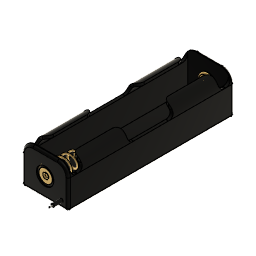
18650 battery holder (Autodesk Fusion 360 design; units mm, degrees)
Autodesk Fusion 360 part; units mm, degrees
note: some values were not read from the file. Set by a fixed rule: which face or edge a step refers to.
sketch "Esquisse1" plane through (0, 0, 0) normal (0, 1, 0) x (1, 0, 0)
  line L0 (-10.6, 9.1) -> (10.6, 9.1)
  line L1 (10.6, 9.1) -> (10.6, -4.1)
  line L2 (5.6, -9.1) -> (-5.6, -9.1)
  line L3 (-10.6, -4.1) -> (-10.6, 9.1)
  line L4 (-10.6, 9.1) -> (10.6, -9.1) construction
  line L5 (10.6, 9.1) -> (-10.6, -9.1) construction
  arc A0 (-10.6, -4.1) -> (-5.6, -9.1) centre (-5.6, -4.1) ccw
  arc A1 (5.6, -9.1) -> (10.6, -4.1) centre (5.6, -4.1) ccw
  dimension "d1" = 21.2
  dimension "d2" = 18.2
  dimension "d3" = 5
  dimension "d4" = 5
  constraint horizontal L0
  constraint perpendicular L0 L1
  constraint parallel L0 L2
  constraint parallel L1 L3
  constraint coincident L4 origin
  constraint coincident L5 origin
  constraint coincident L5.end L3
  constraint coincident L5.end L2
  constraint tangent L3 A0
  constraint tangent L2 A0
  constraint coincident L4.end L2
  constraint coincident L4.end L1
  constraint tangent L2 A1
  constraint tangent L1 A1
  measures "d1" distance of L0.start L0.end
  measures "d2" distance of L0.end L4.end
  measures "d3" radius of A0
  measures "d4" radius of A1
extrude "Extrusion1" add sketch "Esquisse1" along normal blind 76 makes body 1
fillet "Congé1" radius 1 14 edges at (10.6, 0, -2.5) (9.1355, 0, 7.6355) (0, 0, 9.1) (-9.1355, 0, 7.6355) (-10.6, 0, -2.5) (0, 0, -9.1) (10.6, 38, -9.1) (-10.6, 38, -9.1) (-10.6, 76, -2.5) (-9.1355, 76, 7.6355) (0, 76, 9.1) (9.1355, 76, 7.6355) (10.6, 76, -2.5) (0, 76, -9.1) on bodies 1
shell "Coque1" thickness 1.3 removed faces 0 bodies 1
sketch "Esquisse2" plane through (10.6, 0, 0) normal (1, 0, 0) x (0, 1, 0)
  line L0 (75, -8.1) -> (75, 4.1)
  line L1 (75, 4.1) -> (1, 4.1)
  line L2 (1, 4.1) -> (1, -8.1)
  line L3 (1, -8.1) -> (75, -8.1)
  line L4 (38, -8.1) -> (38, 4.1) construction
  line L5 (38, 4.1) -> (27.4849, 4.1)
  line L6 (27.4849, 4.1) -> (27.4849, 10)
  line L7 (27.4849, 10) -> (38, 10)
  line L8 (38, 10) -> (38, 4.1)
  line L9 (1.3, 4.1) -> (6.8127, 4.1)
  line L10 (6.8127, 4.1) -> (6.8127, 10)
  line L11 (6.8127, 10) -> (1.3, 10)
  line L12 (1.3, 10) -> (1.3, 4.1)
  line L13 (69.1873, 10) -> (74.7, 10)
  line L14 (69.1873, 4.1) -> (69.1873, 10)
  line L15 (74.7, 10) -> (74.7, 4.1)
  line L16 (74.7, 4.1) -> (69.1873, 4.1)
  line L17 (38, 4.1) -> (48.5151, 4.1)
  line L18 (48.5151, 4.1) -> (48.5151, 10)
  line L19 (48.5151, 10) -> (38, 10)
  line L20 (38, 10) -> (38, 4.1)
  line L21 (0, 4.1) -> (0, 8.1)
  dimension "d17" = 1.3
  constraint midpoint L3 L4.start
  constraint midpoint L1 L4.end
  constraint horizontal L5
  constraint vertical L6
  constraint horizontal L7
  constraint vertical L8
  constraint horizontal L9
  constraint vertical L10
  constraint horizontal L11
  constraint vertical L12
  constraint symmetric L5.start L4 L8.end
  constraint symmetric L4 L5.end L17.end
  constraint symmetric L4 L6.end L18.end
  constraint symmetric L4 L7.end L8.start
  constraint symmetric L4 L9.start L15.end
  constraint symmetric L4 L9.end L14.start
  constraint symmetric L4 L10.end L13.start
  constraint symmetric L4 L11.end L13.end
  constraint coincident L1 L9.start
  measures "d17" distance of L12 L21
extrude "Extrusion2" cut sketch "Esquisse2" against normal through all contours L1 L13 L14 L15 L16 | L1 L9 L10 L11 L12 | L1 L8 L17 L18 L19 L20 | L1 L5 L6 L7 L8 L20 bodies 1
extrude "Extrusion3" cut 2 faces at (1.8667, 13.7034, 9.1) (1.8667, 55.4058, 9.1) along direction (0, 0, 1) up to surface end surface through (5.6, 0, 7.8) normal (0, 0, -1) offset 0 on bodies 1 bodies 1
fillet "Congé2" radius 2.5 4 edges at (9.95, 6.8127, 4.1) (5.6, 6.8127, 8.45) (9.95, 48.5151, 4.1) (5.6, 48.5151, 8.45) on bodies 1
fillet "Congé2" radius 2.5 4 edges at (9.95, 27.4849, 4.1) (5.6, 27.4849, 8.45) (9.95, 69.1873, 4.1) (5.6, 69.1873, 8.45) on bodies 1
fillet "Congé2" radius 2.5 2 edges at (9.95, 1.3, 4.1) (9.95, 74.7, 4.1) on bodies 1
mirror "Symétrie miroir3" about plane through (0, 0, 0) normal (1, 0, 0) of "Congé2"
hole "Perçage1" at (0, 38, -7.8) direction (0, 0, -1) diameter 3.3 end through all bodies 1
hole "Perçage2" at (0, 76, -0.1627) direction (0, -1, 0) diameter 3 depth 1.3 tip angle 180 counterbore diameter 8 counterbore depth 0.5 bodies 1
hole "Perçage3" at (0, 0, -0.1627) direction (0, 1, 0) diameter 3 depth 1.3 tip angle 180 counterbore diameter 8 counterbore depth 0.5 bodies 1
sketch "Esquisse3" plane through (0, 0, 0) normal (0, -1, 0) x (1, 0, 0)
  line L0 (9.6, -8.1) -> (9.6, 4.1)
  arc A0 (9.6, 4.1) -> (5.6, 8.1) centre (5.6, 4.1) ccw
  line L1 (5.6, 8.1) -> (-5.6, 8.1)
  arc A1 (-5.6, 8.1) -> (-9.6, 4.1) centre (-5.6, 4.1) ccw
  line L2 (-9.6, 4.1) -> (-9.6, -8.1)
  line L3 (-9.6, -8.1) -> (9.6, -8.1)
  circle A2 centre (7.4787, -5.9787) radius 0.75
  circle A3 centre (7.4787, -5.9787) radius 0.25
  line L4 (9.6, -8.1) -> (7.4787, -5.9787) construction
  circle A4 centre (0, -0.1627) radius 4
  dimension "d35" = 1.5
  dimension "d36" = 0.5
  dimension "d37" = 45
  dimension "d38" = 3
  constraint concentric A2 A3
  constraint coincident L0.start L3.end
  constraint coincident A2.centre A3.centre
  measures "d35" diameter of A2
  measures "d36" diameter of A3
  measures "d37" angle of L3 L4
  measures "d38" distance of A2.centre L0.start
extrude "Extrusion4" add sketch "Esquisse3" along normal blind 4 contours A2 | A3 bodies 1
extrude "Extrusion5" add sketch "Esquisse3" along normal blind 5.5 contours A3 bodies 1
sketch "Esquisse4" plane through (0, 76, 0) normal (0, 1, 0) x (-1, 0, 0)
  line L0 (-9.6, -8.1) -> (9.6, -8.1)
  line L1 (9.6, -8.1) -> (9.6, 4.1)
  arc A0 (9.6, 4.1) -> (5.6, 8.1) centre (5.6, 4.1) ccw
  line L2 (5.6, 8.1) -> (-5.6, 8.1)
  arc A1 (-5.6, 8.1) -> (-9.6, 4.1) centre (-5.6, 4.1) ccw
  line L3 (-9.6, 4.1) -> (-9.6, -8.1)
  circle A2 centre (7.4787, -5.9787) radius 0.75
  circle A3 centre (7.4787, -5.9787) radius 0.25
  line L4 (9.6, -8.1) -> (7.4787, -5.9787) construction
  circle A4 centre (0, -0.1627) radius 4
  dimension "d43" = 1.5
  dimension "d44" = 0.5
  dimension "d45" = 45
  dimension "d46" = 3
  constraint concentric A2 A3
  constraint coincident L0.end L1.start
  constraint coincident A2.centre A3.centre
  measures "d43" diameter of A2
  measures "d44" diameter of A3
  measures "d45" angle of L0 L4
  measures "d46" distance of A2.centre L0.end
extrude "Extrusion6" add sketch "Esquisse4" along normal blind 4 contours A2 | A3 bodies 1
extrude "Extrusion7" add sketch "Esquisse4" along normal blind 5.5 contours A3 bodies 1
coil "SpirePrimitive1" add diameter 8 section circle size 0.8 on centre turns 5 pitch 3 right hand placed x (-1, 0, 0) y (0, 0, 1) z (0, 1, 0) at (0, 1.3, 0) taper angle -5 bodies 1
sketch "Esquisse6" plane through (0, 0, 0) normal (1, 0, 0) x (0, 1, 0)
  line L0 (75.5, 1.3373) -> (75.5, -1.6627) construction
  line L1 (74.7, -1.6627) -> (74.7, 1.3373) construction
  line L2 (74.6808, 3.8373) -> (74.6808, 1.3025)
  line L3 (74.7, -0.1627) -> (75.5, -0.1627)
  line L4 (75.1, -0.1627) -> (75.1, 1.3025) construction
  line L5 (74.6808, 3.8373) -> (73.6808, 3.8373)
  line L6 (73.6808, 3.8373) -> (73.6808, 0.6095)
  line L7 (73.6808, 0.6095) -> (75.1, 0.6095)
  line L8 (74.6808, 1.3025) -> (75.1, 1.3025)
  line L9 (75.1, 1.3025) -> (75.5352, 1.3025)
  line L10 (75.5352, 1.3025) -> (75.5352, 2.9)
  line L11 (75.5352, 2.9) -> (75.7832, 2.9)
  line L12 (75.7832, 2.9) -> (75.7832, 0.6095)
  line L13 (75.7832, 0.6095) -> (75.1, 0.6095)
  dimension "d60" = 1
  dimension "d61" = 4
  constraint parallel L0 L2
  constraint midpoint L1 L3.start
  constraint midpoint L0 L3.end
  constraint midpoint L3 L4.start
  constraint perpendicular L3 L4
  constraint perpendicular L2 L5
  constraint perpendicular L5 L6
  constraint coincident L4 L7.end
  constraint perpendicular L4 L7
  constraint perpendicular L4 L8
  constraint perpendicular L0 L9
  constraint perpendicular L9 L10
  constraint perpendicular L10 L11
  constraint perpendicular L11 L12
  constraint collinear L7 L13
  measures "d60" distance of L2.start L5.end
  measures "d61" distance of L3 L5
revolve "Révolution1" add sketch "Esquisse6" angle 360 about axis through (0, 74.7, -0.1627) along (0, 1, 0) separate body makes body 2
fillet "Congé3" radius 0.75 2 edges at (-0.7199, 73.6808, 0.1165) (-3.7293, 73.6808, 1.2838) on bodies 2
fillet "Congé3" radius 0.5 1 edges at (-0.7199, 75.7832, 0.1165) on bodies 2
ref_plane "Plan de construction2" through (0, 38, 0) normal (0, -1, 0) x (-1, 0, 0)
mirror "Symétrie miroir4" about plane through (0, 38, 0) normal (0, -1, 0) of bodies 2 makes body 3
